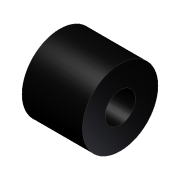
# Autodesk Inventor part: Shovel_CylinderMountSpacer
Saved by Autodesk Inventor 2012 (Build 160160000, 160)
## iProperties
Created: 2013-02-01
Part Number: Shovel_CylinderMountSpacer
Material: Aluminum-6061-AHC
Document SubType Name: Modeling
Designer: JesseK
Density: 2.71 g/cm^3
Mass: 5.71355 g
Surface Area: 12.1977 cm^2
Volume: 2.10832 cm^3
Author: JesseK
Autodesk Inventor part; units mm, degrees
ref_plane "YZ Plane" through (0, 0, 0) normal (1, 0, 0) x (0, 1, 0)
ref_plane "XZ Plane" through (0, 0, 0) normal (0, 1, 0) x (-1, 0, 0)
ref_plane "XY Plane" through (0, 0, 0) normal (0, 0, 1) x (1, 0, 0)
sketch "Sketch1" plane through (0, 0, 0) normal (1, 0, 0) x (0, 1, 0)
  circle A0 centre (0, 0) radius 3.1877
  circle A1 centre (0, 0) radius 7.9375
  dimension "d0" = 6.3754
  dimension "d1" = 15.875
  constraints: 2 centre point, 2 coincident
  measures "d0" diameter of A0
  measures "d1" diameter of A1
extrude "Extrusion1" add sketch "Sketch1" along normal blind 12.7
body "Solid1"
